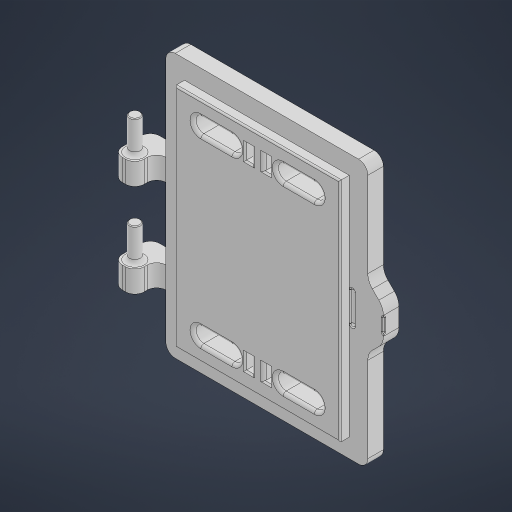
# Autodesk Inventor part: 케이스 베이스
Saved by Autodesk Inventor 2024 (Build 280153000, 153)
## iProperties
Created: 2023-12-08
Part Number: 케이스 베이스
Material: 일반
Document SubType Name: Modeling
Designer: KBU
Density: 1 g/cm^3
Appearance: 기본값
Author: KBU
Autodesk Inventor part; units mm, degrees
ref_plane "YZ Plane" through (0, 0, 0) normal (1, 0, 0) x (0, 1, 0)
ref_plane "XZ Plane" through (0, 0, 0) normal (0, 1, 0) x (-1, 0, 0)
ref_plane "XY Plane" through (0, 0, 0) normal (0, 0, 1) x (1, 0, 0)
sketch "스케치1" plane through (0, 0, 0) normal (0, 0, 1) x (1, 0, 0)
  line L0 (-32.5, -42.5) -> (32.5, -42.5)
  line L1 (32.5, -42.5) -> (32.5, 42.5)
  line L2 (32.5, 42.5) -> (-32.5, 42.5)
  line L3 (-32.5, 42.5) -> (-32.5, -42.5)
  line L4 (-32.5, -42.5) -> (32.5, 42.5) construction
  line L5 (32.5, -42.5) -> (-32.5, 42.5) construction
  point P0 (0, 0)
  dimension "d0" = 65
  dimension "d1" = 85
  constraints: 12 end point, 2 midpoint, 2 parallel, 1 horizontal, 1 perpendicular
  measures "d0" distance of L1.end L2.end
  measures "d1" distance of L2.end L0.start
extrude "돌출1" add sketch "스케치1" along normal blind 5
sketch "스케치2" plane through (0, 0, 5) normal (0, 0, 1) x (1, 0, 0)
  line L0 (32.5, -42.5) -> (32.5, 42.5) projected
  line L1 (32.5, 42.5) -> (-32.5, 42.5) projected
  line L2 (-32.5, 42.5) -> (-32.5, -42.5) projected
  line L3 (-32.5, -42.5) -> (32.5, -42.5) projected
  line L4 (-26.5, -36.5) -> (-26.5, 36.5)
  line L5 (-26.5, 36.5) -> (26.5, 36.5)
  line L6 (26.5, 36.5) -> (26.5, -36.5)
  line L7 (26.5, -36.5) -> (-26.5, -36.5)
  point P0 (0, 0)
  dimension "d4" = 6
  constraints: 8 end point, 3 other
  measures "d4" distance between parallel lines of L2 L4
extrude "돌출2" add sketch "스케치2" along normal blind 3 contours L4 L5 L6 L7
sketch "스케치3" plane through (-32.5, -42.5, 0) normal (-1, 0, 0) x (0, 0, 1)
  line L0 (0, 85) -> (0, 0) projected
  line L1 (0, 24.5) -> (12, 24.5)
  line L2 (12, 24.5) -> (12, 17.5)
  line L3 (12, 17.5) -> (0, 17.5)
  line L4 (0, 17.5) -> (0, 24.5)
  line L5 (0, 0) -> (5, 0) projected
  line L6 (0, 54.5) -> (12, 54.5)
  line L7 (12, 54.5) -> (12, 47.5)
  line L8 (12, 47.5) -> (0, 47.5)
  line L9 (0, 47.5) -> (0, 54.5)
  point P0 (0, 42.5)
  point P1 (0, 17.5)
  point P2 (2.5, 0)
  point P3 (0, 47.5)
  dimension "d7" = 7
  dimension "d10" = 17.5
  dimension "d11" = 12
  dimension "d16" = 12
  dimension "d17" = 7
  dimension "d18" = 23
  constraints: 16 end point, 4 parallel, 2 horizontal, 2 perpendicular, 2 point on line, 1 midpoint
  measures "d7" distance between parallel lines of L3 L1
  measures "d10" distance from line of point (2.5, 0) L3
  measures "d11" distance between parallel lines of L0 L2
  measures "d16" distance of L6.start L6.end
  measures "d17" distance between parallel lines of L8 L6
  measures "d18" distance between parallel lines of L1 L8
extrude "돌출3" add sketch "스케치3" along normal blind 10
sketch "스케치4" plane through (-32.5, -25, 12) normal (0, 0, 1) x (1, 0, 0)
  line L0 (0, 0) -> (0, 7) projected
  line L1 (0, 7) -> (-10, 7) projected
  line L2 (-10, 0) -> (-10, 7) projected
  line L3 (0, 0) -> (-10, 0) projected
  line L4 (0, 7) -> (-3, 7)
  line L5 (-3, 7) -> (-3, 0)
  line L6 (-3, 0) -> (0, 0)
  line L7 (0, 0) -> (0, 7)
  line L8 (0, 67.5) -> (0, 37) projected
  line L9 (0, 30) -> (-10, 30) projected
  line L10 (0, 37) -> (-3, 37)
  line L11 (-3, 37) -> (-3, 30)
  line L12 (-3, 30) -> (0, 30)
  line L13 (0, 30) -> (0, 37)
  line L14 (-10, 30) -> (-10, 37) projected
  point P0 (32.5, 25)
  point P1 (-3, 7)
  point P2 (-3, 33.5)
  dimension "d12" = 7
  dimension "d19" = 7
  constraints: 16 end point, 4 parallel, 2 horizontal, 2 perpendicular, 2 point on line, 1 midpoint
  measures "d12" distance between parallel lines of L5 L2
  measures "d19" distance from line of L14 point (-3, 33.5)
extrude "돌출4" cut sketch "스케치4" against normal blind 7 contours L3 L5 L1 L0 | L9 L11 L10 L13
sketch "스케치5" plane through (-32.5, -18, 5) normal (0, 1, 0) x (1, 0, 0)
  circle A0 centre (-6.5, -3.5) radius 1.75
  point P0 (32.5, 5)
  dimension "d20" = 3.5
  constraints: 1 centre point
  measures "d20" diameter of A0
extrude "돌출5" add sketch "스케치5" along normal blind 10.5
sketch "스케치6" plane through (-32.5, 12, 5) normal (0, 1, 0) x (1, 0, 0)
  circle A0 centre (-6.5, -3.5) radius 1.75
  line L0 (-3, -7) -> (-10, -7) projected
  line L1 (-3, -7) -> (-3, 0) projected
  point P0 (32.5, 5)
  dimension "d23" = 3.5
  dimension "d27" = 3.5
  dimension "d28" = 3.5
  constraints: 1 centre point
  measures "d23" diameter of A0
  measures "d27" distance from line of L1 A0.centre
  measures "d28" distance from line of A0.centre L0
extrude "돌출6" add sketch "스케치6" along normal blind 10.5
fillet "모깎기1" radius 3 8 edges at (-42.5, -21.5, 12) (-35.5, -21.5, 12) (-42.5, -21.5, 0) (-35.5, -21.5, 5) (-35.5, 8.5, 5) (-35.5, 8.5, 12) (-42.5, 8.5, 12) (-42.5, 8.5, 0)
fillet "모깎기2" radius 3 4 edges at (32.5, 42.5, 2.5) (-32.5, 42.5, 2.5) (-32.5, -42.5, 2.5) (32.5, -42.5, 2.5)
fillet "모깎기3" radius 0.5 4 edges at (26.5, 0, 8) (0, -36.5, 8) (-26.5, 0, 8) (0, 36.5, 8)
sketch "스케치7" plane through (0, 0, 5) normal (0, 0, 1) x (1, 0, 0)
  line L0 (26.5, 36.5) -> (26.5, -36.5) projected
  line L1 (27.5, -4.6426) -> (27.5, 4.6426) construction
  line L2 (28.2, -4.6426) -> (28.2, 4.6426)
  line L3 (26.8, 4.6426) -> (26.8, -4.6426)
  arc A0 (26.8, -4.6426) -> (28.2, -4.6426) centre (27.5, -4.6426) ccw
  arc A1 (28.2, 4.6426) -> (26.8, 4.6426) centre (27.5, 4.6426) ccw
  line L4 (27.5, 6.6849) -> (27.5, -6.9457)
  point P0 (0, 0)
  point P1 (27.5, 0)
  point P2 (27.5, 5.3426)
  point P3 (27.5, -5.3426)
  dimension "d31" = 0.7
  dimension "d32" = 1
  constraints: 10 end point, 4 point on circle, 4 tangent, 2 centre point, 2 vertical, 1 midpoint, 1 parallel, 1 point on line
  measures "d31" radius of A1
  measures "d32" distance from line of L0 point (27.5, 0)
revolve "회전1" cut sketch "스케치7" angle 360 about axis through (27.5, 6.6849, 5) along (0, -1, 0) contours A0 L4 A1 L2
fillet "모깎기4" radius 0.4 6 edges at (27.995, 5.1376, 5) (27.005, 5.1376, 5) (28.2, 0, 5) (26.8, 0, 5) (27.005, -5.1376, 5) (27.995, -5.1376, 5)
fillet "모깎기5" radius 1.25 2 edges at (-40.75, -18, 8.5) (-40.75, 12, 8.5)
chamfer "모따기1" distance 0.25 angle 45 2 edges at (-40.75, 22.5, 8.5) (-40.75, -7.5, 8.5)
sketch "스케치8" plane through (0, 0, 0) normal (0, 0, -1) x (-1, 0, 0)
  line L0 (-32.5, -39.5) -> (-32.5, 39.5) projected
  line L1 (-27.5, -5) -> (-37.5, -5)
  line L2 (-37.5, -5) -> (-37.5, 5)
  line L3 (-37.5, 5) -> (-27.5, 5)
  line L4 (-27.5, 5) -> (-27.5, -5)
  line L5 (-27.5, -5) -> (-37.5, 5) construction
  line L6 (-37.5, -5) -> (-27.5, 5) construction
  line L7 (-37.5, 5) -> (-32.5, 10)
  line L8 (-37.5, -5) -> (-32.5, -10)
  point P0 (0, 0)
  point P1 (-32.5, 0)
  dimension "d39" = 10
  dimension "d40" = 10
  dimension "d41" = 20
  constraints: 16 end point, 3 midpoint, 2 parallel, 2 perpendicular, 2 point on line, 1 horizontal
  measures "d39" distance of L2.end L3.end
  measures "d40" distance of L1.end L2.end
  measures "d41" distance of L7.end L8.end
extrude "돌출7" add sketch "스케치8" against normal up to surface (5 mm away) contours L8 L1 L0 | L1 L2 L3 L0 | L3 L7 L0
fillet "모깎기6" radius 5 4 edges at (32.5, -10, 2.5) (37.5, -5, 2.5) (37.5, 5, 2.5) (32.5, 10, 2.5)
sketch "스케치9" plane through (37.5, -2.9289, 0) normal (1, 0, 0) x (0, 0, -1)
  line L0 (-5, 5.8579) -> (-5, 0) projected
  line L1 (-5, 0.9289) -> (-5, 4.9289) construction
  line L2 (-4.5, 0.9289) -> (-4.5, 4.9289)
  line L3 (-5.5, 4.9289) -> (-5.5, 0.9289)
  arc A0 (-5.5, 0.9289) -> (-4.5, 0.9289) centre (-5, 0.9289) ccw
  arc A1 (-4.5, 4.9289) -> (-5.5, 4.9289) centre (-5, 4.9289) ccw
  line L4 (-5, 5.8579) -> (-5, 0)
  line L5 (-4.7455, -1.7137) -> (-4.7455, 7.5716) projected
  point P0 (0, 2.9289)
  point P1 (-5, 2.9289)
  point P2 (-5, 5.4289)
  point P3 (-5, 0.4289)
  dimension "d45" = 0.5
  dimension "d46" = 4
  constraints: 10 end point, 4 point on circle, 4 tangent, 2 centre point, 2 midpoint, 2 parallel, 1 point on line
  measures "d45" radius of A1
  measures "d46" distance of L2.start L2.end
revolve "회전2" cut sketch "스케치9" angle 360 about axis through (37.5, 2.9289, 5) along (0, -1, 0) contours A1 L5 A0 L0 | A1 L2 A0 L5
fillet "모깎기7" radius 0.3 6 edges at (37.5, -2.3536, 4.6464) (37.5, 2.3536, 4.6464) (37.5, 0, 4.5) (37.1464, 2.3536, 5) (37.1464, -2.3536, 5) (37, 0, 5)
sketch "스케치10" plane through (0, 0, 8) normal (0, 0, 1) x (1, 0, 0)
  line L0 (-18.25, -29.25) -> (-8.25, -29.25) construction
  line L1 (-18.25, -31.75) -> (-8.25, -31.75)
  line L2 (-8.25, -26.75) -> (-18.25, -26.75)
  arc A0 (-18.25, -26.75) -> (-18.25, -31.75) centre (-18.25, -29.25) ccw
  arc A1 (-8.25, -31.75) -> (-8.25, -26.75) centre (-8.25, -29.25) ccw
  line L3 (-26.5, 36.5) -> (-26.5, -36.5) projected
  line L4 (-26.5, -36.5) -> (26.5, -36.5) projected
  line L5 (0, 0) -> (0, -43.4642)
  line L6 (18.25, -29.25) -> (8.25, -29.25) construction
  line L7 (18.25, -31.75) -> (8.25, -31.75)
  line L8 (8.25, -26.75) -> (18.25, -26.75)
  arc A2 (18.25, -31.75) -> (18.25, -26.75) centre (18.25, -29.25) ccw
  arc A3 (8.25, -26.75) -> (8.25, -31.75) centre (8.25, -29.25) ccw
  line L9 (-38.2578, 0) -> (54.5132, 0)
  line L10 (-18.25, 29.25) -> (-8.25, 29.25) construction
  line L11 (-18.25, 31.75) -> (-8.25, 31.75)
  line L12 (-8.25, 26.75) -> (-18.25, 26.75)
  arc A4 (-18.25, 31.75) -> (-18.25, 26.75) centre (-18.25, 29.25) ccw
  arc A5 (-8.25, 26.75) -> (-8.25, 31.75) centre (-8.25, 29.25) ccw
  arc A6 (18.25, 26.75) -> (18.25, 31.75) centre (18.25, 29.25) ccw
  line L13 (18.25, 31.75) -> (8.25, 31.75)
  line L14 (18.25, 29.25) -> (8.25, 29.25) construction
  line L15 (8.25, 26.75) -> (18.25, 26.75)
  arc A7 (8.25, 31.75) -> (8.25, 26.75) centre (8.25, 29.25) ccw
  line L16 (-4, -26.75) -> (-2, -26.75)
  line L17 (-2, -26.75) -> (-2, -31.75)
  line L18 (-2, -31.75) -> (-4, -31.75)
  line L19 (-4, -31.75) -> (-4, -26.75)
  line L20 (4, -26.75) -> (2, -26.75)
  line L21 (2, -26.75) -> (2, -31.75)
  line L22 (2, -31.75) -> (4, -31.75)
  line L23 (4, -31.75) -> (4, -26.75)
  line L24 (-4, 26.75) -> (-2, 26.75)
  line L25 (-2, 26.75) -> (-2, 31.75)
  line L26 (-2, 31.75) -> (-4, 31.75)
  line L27 (-4, 31.75) -> (-4, 26.75)
  line L28 (4, 26.75) -> (2, 26.75)
  line L29 (4, 31.75) -> (4, 26.75)
  line L30 (2, 26.75) -> (2, 31.75)
  line L31 (2, 31.75) -> (4, 31.75)
  point P0 (-13.25, -29.25)
  point P1 (13.25, -29.25)
  point P2 (-13.25, 29.25)
  point P3 (13.25, 29.25)
  dimension "d49" = 13.25
  dimension "d50" = 10
  dimension "d51" = 26.5
  dimension "d52" = 7.25
  dimension "d53" = 2.5
  dimension "d56" = 5
  dimension "d57" = 2
  dimension "d58" = 4
  constraints: 68 end point, 33 symmetric about line, 16 point on circle, 8 centre point, 4 tangent, 3 horizontal, 3 parallel, 1 collinear, 1 midpoint, 1 perpendicular, 1 vertical, 6 other
  measures "d49" distance from line of L3 point (-13.25, -29.25)
  measures "d50" distance of L2.start L2.end
  measures "d51" distance from line of L3 L5.start
  measures "d52" distance from line of L4 point (-13.25, -29.25)
  measures "d53" radius of A1
  measures "d56" distance of L16.end L17.end
  measures "d57" distance of L16.start L16.end
  measures "d58" diameter of L17 L5
extrude "돌출8" cut sketch "스케치10" against normal up to surface (8 mm away) contours A0 L2 A1 L1 | L7 A3 L8 A2 | L11 A5 L12 A4 | L15 A7 L13 A6 | L16 L17 L18 L19 | L23 L22 L21 L20 | L27 L26 L25 L24 | L28 L30 L31 L29
fillet "모깎기8" radius 1 20 edges at (-20.75, -29.25, 8) (-13.25, -26.75, 8) (-5.75, -29.25, 8) (-13.25, -31.75, 8) (13.25, -26.75, 8) (20.75, -29.25, 8) (13.25, -31.75, 8) (5.75, -29.25, 8) (-20.75, 29.25, 8) (-13.25, 31.75, 8) (-5.75, 29.25, 8) (-13.25, 26.75, 8) (13.25, 31.75, 8) (20.75, 29.25, 8) (13.25, 26.75, 8) (5.75, 29.25, 8) (-2, 29.25, 8) (2, 29.25, 8) (-2, -29.25, 8) (2, -29.25, 8)
chamfer "모따기2" distance 0.5 angle 45 12 edges at (-3, -26.75, 8) (-4, -29.25, 8) (-3, -31.75, 8) (3, -26.75, 8) (4, -29.25, 8) (3, -31.75, 8) (-3, 26.75, 8) (-4, 29.25, 8) (-3, 31.75, 8) (3, 31.75, 8) (4, 29.25, 8) (3, 26.75, 8)
equation "\"d16\" = d11"
equation "\"d17\" = d7"
equation "\"d19\" = d12"
